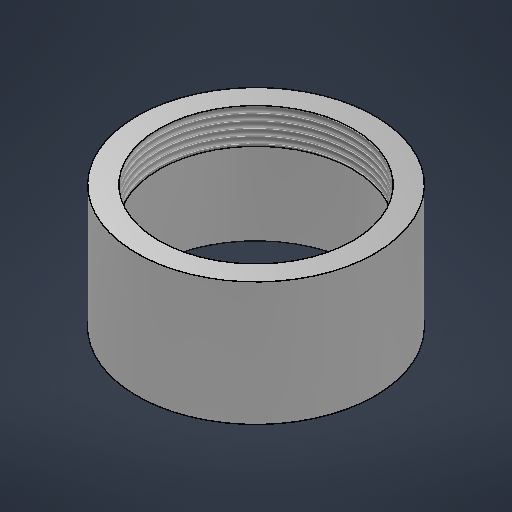
# Autodesk Inventor part: Top Nut
Saved by Autodesk Inventor 2026 (Build 300175050, 175E)
## iProperties
Created: 2025-06-28
Part Number: Top Nut
Material: ABS Plastic
Document SubType Name: Modeling
Designer: Joshua Eah
Density: 1.06 g/cm^3
Appearance: Anodized - Light Gray
Author: Joshua Eah
Autodesk Inventor part; units mm, degrees
ref_plane "YZ Plane" through (0, 0, 0) normal (1, 0, 0) x (0, 1, 0)
ref_plane "XZ Plane" through (0, 0, 0) normal (0, 1, 0) x (-1, 0, 0)
ref_plane "XY Plane" through (0, 0, 0) normal (0, 0, 1) x (1, 0, 0)
sketch "Sketch1" plane through (0, 0, 0) normal (0, 1, 0) x (-1, 0, 0)
  circle A0 centre (0, 0) radius 13.5
  circle A1 centre (0, 0) radius 12
  circle A2 centre (0, 0) radius 11
  dimension "d0" = 27
  dimension "d1" = 24
  dimension "d4" = 22
  constraints: 3 centre point, 3 coincident
  measures "d0" diameter of A0
  measures "d1" diameter of A1
  measures "d4" diameter of A2
extrude "Extrusion1" add sketch "Sketch1" along normal blind 14 contours A0 | A1
extrude "Extrusion2" cut sketch "Sketch1" along normal blind 10 contours A1
thread "Thread1" size "M22x0.75" class "6H" standard "ANSI Metric M Profile" full length
body "Solid1"
